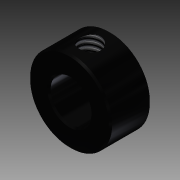
# Autodesk Inventor part: Misc_ShaftCollar_Ruland_SC-6-F
Saved by Autodesk Inventor 2014 (Build 180170000, 170)
## iProperties
Category: Miscellaneous
Company: Autodesk Inc.
Created: 2012-12-03
Part Number: Misc_ShaftCollar_Ruland_SC-6-F
Document SubType Name: Modeling
Designer: Autodesk Inc.
Density: 7.87 g/cm^3
Material: Steel, Carbon
Appearance: Smooth - Black
Author: Autodesk Inc.
Autodesk Inventor part; units mm, degrees
note: some values were not read from the file. Chosen so that the rebuilt part matches the saved one: direction of "Hole1".
ref_plane "YZ Plane" through (0, 0, 0) normal (1, 0, 0) x (0, 1, 0)
ref_plane "XY Plane" through (0, 0, 0) normal (0, 0, 1) x (1, 0, 0)
sketch "Sketch1" plane through (0, 0, 0) normal (0, 0, 1) x (1, 0, 0)
  circle A0 centre (0, 0) radius 9.525
  dimension "d0" = 19.05
  constraints: 1 centre point, 1 coincident
  measures "d0" diameter of A0
extrude "Extrusion1" add sketch "Sketch1" against normal blind 9.525
sketch "Sketch2" plane through (0, 0, 0) normal (0, 0, 1) x (1, 0, 0)
  circle A0 centre (0, 0) radius 9.525 projected
  circle A1 centre (0, 0) radius 4.7625
  dimension "d3" = 9.525
  constraints: 1 centre point, 1 coincident
  measures "d3" diameter of A1
extrude "Extrusion2" cut sketch "Sketch2" against normal up to next contours A1
chamfer "Chamfer1" distance 0.3969 angle 45 4 edges at (-9.525, 0, 0) (-9.525, 0, -9.525) (-4.7625, 0, 0) (-4.7625, 0, -9.525)
ref_plane "Work Plane1" through (0, 9.525, 0) normal (0, 1, 0) x (-1, 0, 0)
sketch "Sketch3" plane through (0, 9.525, 0) normal (0, 1, 0) x (-1, 0, 0)
  line L0 (9.1281, -9.525) -> (-9.1281, -9.525) projected
  line L1 (9.525, -0.3969) -> (9.525, -9.1281) projected
  point P0 (0, 0)
  point P1 (0, -4.7625)
  point P2 (0, -9.525)
  point P3 (9.525, -4.7625)
  constraints: 2 midpoint, 1 horizontal alignment, 1 vertical alignment
hole "Hole1" at (0, 9.525, -4.7625) direction (0, -1, 0) diameter 4.9784 end up to surface thread size "1/4-20 UNC" class "2B" standard "ANSI Unified Screw Threads"
body "Solid1"
